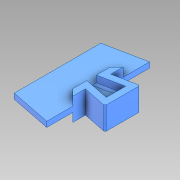
# Autodesk Inventor part: MaleDoubleSide
Saved by Autodesk Inventor 2021.4 (Build 254397000, 397)
## iProperties
Created: 2021-02-11
Part Number: MaleDoubleSide
Material: ABS プラスチック
Document SubType Name: Modeling
Designer: kumagai
Density: 1.06 g/cm^3
Appearance: 滑らか - 青
cp: 0.000 mm
ConnectorLength: 15.000 mm
RailWidth: 38.000 mm
JointFH: 9.500 mm
PrinterOffset: 0.000 mm
StraightLength: 215.000 mm
OuterWall: 2.000 mm
InnerWall: 2.400 mm
InsideWidth: 18.600 mm
RailHeight: 8.400 mm
RailDepth: 3.200 mm
JointMW1: 13.000 mm
JointMW2: 9.400 mm
JointMH: 9.000 mm
JointFW1: 13.300 mm
JointFW2: 9.600 mm
SupportGap: 0.200 mm
SupportRib: 0.650 mm
d111: 9.000 mm
d112: 2.400 mm
d113: 18.600 mm
d114: 38.000 mm
d115: 2.000 mm
d116: 13.000 mm
d117: 9.400 mm
d119: 0.000 mm
d118: 0.000 mm
d144: 0.000 mm
d143: 0.000 mm
d179: 0.500 mm
Author: kumagai
Autodesk Inventor part; units mm, degrees
ref_plane "YZ Plane" through (0, 0, 0) normal (1, 0, 0) x (0, 1, 0)
ref_plane "BackFace" through (0, -1, 0) normal (0, 1, 0) x (-1, 0, 0)
ref_plane "BottomFace" through (0, -4.2, 0) normal (0, 1, 0) x (-1, 0, 0)
sketch "FemaleOutline" plane through (0, 0, 0) normal (0, 1, 0) x (-1, 0, 0)
  line L0 (0, -26.6) -> (0, 26.6) projected
  line L1 (-3, 0) -> (18, 0) projected
  line L2 (0.4908, -4.8956) -> (9.5, -6.65)
  line L3 (9.5, -6.65) -> (9.5, 6.65)
  line L4 (9.5, 6.65) -> (0.4908, 4.8956)
  line L5 (0, -19) -> (0, -5.3)
  line L6 (0, 5.3) -> (0, 19)
  line L7 (2.4, -6.9) -> (11.5, -6.9)
  line L8 (11.5, -6.9) -> (11.5, 6.9)
  line L9 (11.5, 6.9) -> (2.4, 6.9)
  line L10 (2.4, -6.9) -> (0, -9.3)
  line L11 (2.4, 6.9) -> (0, 9.3)
  line L12 (15, -16) -> (15, 16)
  line L13 (15, 16) -> (0, 19)
  line L14 (15, -16) -> (0, -19)
  line L15 (0.4908, 4.8956) -> (0, 5.3)
  line L16 (0.4908, -4.8956) -> (0, -5.3)
  point P0 (0, 0)
  point P1 (0, -4.8)
  point P2 (0, 4.8)
  point P3 (0, 9.3)
  point P4 (0, 4.8)
  point P5 (0, -4.8)
  point P6 (0, -9.3)
  point P7 (0, -5.3)
  point P8 (0, 5.3)
  dimension "d3" = 13.3
  dimension "d5" = 9.6
  dimension "d14" = 2
  dimension "d63" = 2.4
  dimension "d64" = 18.6
  dimension "d65" = 15
  dimension "d74" = 38
  dimension "d75" = 3
  dimension "d93" = 9.5
  dimension "d94" = 2.4
  dimension "d95" = 0.5
  dimension "d96" = 0.5
  dimension "d97" = 0.5
  dimension "d98" = 0.5
  constraints: 30 end point, 6 point on line, 2 collinear, 2 horizontal, 2 vertical, 1 parallel, 1 symmetric about line, 3 other
  measures "d3" distance of L3.end L2.end
  measures "d5" distance of point (0, 4.8) point (0, -4.8)
  measures "d14" distance between parallel lines of L3 L8
  measures "d63" horizontal distance of L10.end L7.start
  measures "d64" distance of L11.end L10.end
  measures "d65" distance between parallel lines of L12 L0
  measures "d74" distance of L5.start L6.end
  measures "d75" vertical distance of L12.end L6.end
  measures "d93" distance between parallel lines of L0 L3
  measures "d94" distance from line of L0 L7.start
  measures "d95" distance of L4.end point (0, 4.8)
  measures "d96" distance of L6.start point (0, 4.8)
  measures "d97" distance of L2.start point (0, -4.8)
  measures "d98" distance of L5.end point (0, -4.8)
sketch "MaleOutline" plane through (0, 0, 0) normal (0, 1, 0) x (-1, 0, 0)
  line L0 (0, -4.7) -> (-8.5097, -6.4019)
  line L1 (-9, -6) -> (-9, 6)
  line L2 (-8.5097, 6.4019) -> (0, 4.7)
  line L3 (0, -19) -> (0, -4.7)
  line L4 (0, 4.7) -> (0, 19)
  line L5 (2.4, -1.7725) -> (-6.6, -3.5725)
  line L6 (-6.6, -3.5725) -> (-6.6, 3.5725)
  line L7 (-6.6, 3.5725) -> (2.4, 1.7725)
  line L8 (2.4, -6.9) -> (2.4, -1.7725)
  line L9 (2.4, 1.7725) -> (2.4, 6.9)
  line L10 (2.4, -6.9) -> (0, -9.3)
  line L11 (2.4, 6.9) -> (0, 9.3)
  line L12 (15, -16) -> (15, 16)
  line L13 (15, 16) -> (0, 19)
  line L14 (15, -16) -> (0, -19)
  line L15 (0, -26.6) -> (0, 26.6) projected
  line L16 (-13.8, 0) -> (19.8, 0) projected
  line L17 (-8.5097, -6.4019) -> (-9, -6)
  line L18 (-9, 6) -> (-8.5097, 6.4019)
  point P0 (-9, -6.5)
  point P1 (-9, 6.5)
  dimension "d99" = 9
  dimension "d100" = 13
  dimension "d101" = 9.4
  dimension "d102" = 2.4
  dimension "d103" = 2.4
  dimension "d104" = 2.4
  dimension "d105" = 2.4
  dimension "d106" = 2.4
  dimension "d107" = 18.6
  dimension "d109" = 38
  dimension "d110" = 3
  dimension "d120" = 15
  dimension "d128" = 0.5
  dimension "d129" = 0.5
  dimension "d130" = 0.5
  dimension "d131" = 0.5
  constraints: 34 end point, 7 point on line, 3 parallel, 2 collinear, 2 vertical, 3 other
  measures "d99" distance between parallel lines of L1 L3
  measures "d100" distance of point (-9, 6.5) point (-9, -6.5)
  measures "d101" distance of L4.start L0.start
  measures "d102" distance between parallel lines of L3 L8
  measures "d103" distance between parallel lines of L1 L6
  measures "d104" distance between parallel lines of L2 L7
  measures "d105" distance between parallel lines of L5 L0
  measures "d106" horizontal distance of L10.end L8.start
  measures "d107" distance of L11.end L10.end
  measures "d109" distance of L3.start L4.end
  measures "d110" vertical distance of L13.start L4.end
  measures "d120" distance between parallel lines of L4 L12
  measures "d128" distance of L0.end point (-9, -6.5)
  measures "d129" distance of L1.start point (-9, -6.5)
  measures "d130" distance of L1.end point (-9, 6.5)
  measures "d131" distance of L2.start point (-9, 6.5)
sketch "DipOutline" plane through (0, -1, 0) normal (0, 1, 0) x (-1, 0, 0)
  line L0 (0, -120.0212) -> (0, 93.8212) projected
  line L1 (-3, 0) -> (18, 0) projected
  line L2 (0, 19) -> (15, 16)
  line L3 (15, 16) -> (15, -16)
  line L4 (15, -16) -> (0, -19)
  line L5 (0, -19) -> (0, 19)
  line L6 (0, 19) -> (0, 4.7)
  line L7 (10.95, -6.3) -> (14.95, -6.3)
  line L8 (14.95, -6.3) -> (14.95, -2.6)
  line L9 (14.95, -2.6) -> (10.95, -2.6)
  line L10 (10.95, -2.6) -> (10.95, -6.3)
  line L11 (14.95, -15.85) -> (14.95, -10.35)
  arc A0 (14.95, -10.35) -> (0, -8.95) centre (0, -89.4723) ccw
  arc A1 (0, -17.25) -> (14.95, -15.85) centre (0, 63.2723) ccw
  line L12 (9.5, 0) -> (9.5, -6.9)
  line L13 (9.5, -6.9) -> (0, -6.9)
  line L14 (0, -8.45) -> (0.5, -8.9516)
  line L15 (0, -17.75) -> (0.5, -17.2484)
  point P0 (0, -17.25)
  point P1 (15, 0)
  point P2 (0, 0)
  point P3 (0, -8.95)
  dimension "d133" = 15
  dimension "d134" = 38
  dimension "d135" = 3
  dimension "d146" = 3.7
  dimension "d147" = 6.3
  dimension "d148" = 2.6
  dimension "d151" = 14.95
  dimension "d152" = 4
  dimension "d153" = 5.5
  dimension "d154" = 8.3
  dimension "d155" = 17.25
  dimension "d160" = 6.9
  dimension "d161" = 9.5
  dimension "d196" = 0.5
  dimension "d197" = 0.5
  dimension "d198" = 0.5
  dimension "d199" = 0.5
  constraints: 28 end point, 8 point on line, 6 point on circle, 5 vertical, 2 centre point, 2 horizontal, 2 line through centre, 2 parallel, 1 collinear, 1 equal radius, 1 other
  measures "d133" distance between parallel lines of L0 L3
  measures "d134" distance of L2.start L4.end
  measures "d135" vertical distance of L2.start L2.end
  measures "d146" distance between parallel lines of L7 L9
  measures "d147" distance between parallel lines of L1 L7
  measures "d148" distance between parallel lines of L1 L9
  measures "d151" distance between parallel lines of L8 L0
  measures "d152" distance between parallel lines of L8 L10
  measures "d153" distance of L11.end L11.start
  measures "d154" distance of A0.end A1.start
  measures "d155" distance from line of L1 A1.start
  measures "d160" distance between parallel lines of L13 L1
  measures "d161" distance between parallel lines of L5 L12
  measures "d196" distance of A0.end L14.start
  measures "d197" distance of L14.end A0.end
  measures "d198" distance of A1.start L15.end
  measures "d199" distance of A1.start L15.start
sketch "DipSupport" plane through (0, -4.2, 0) normal (0, 1, 0) x (-1, 0, 0)
  line L0 (0, -20.94) -> (0, 3.49) projected
  line L1 (-5.0794, 0) -> (17.4132, 0) projected
  line L2 (-1.8662, -13.1) -> (-0.8497, -13.1)
  line L3 (0, -9.95) -> (0, -16.25)
  line L4 (0, -16.25) -> (0.6, -16.25)
  line L5 (0.6, -16.25) -> (0.6, -15.5)
  line L6 (0.6, -14.8486) -> (0.6, -13.35)
  line L7 (0.6, -13.35) -> (13.117, -13.35)
  line L8 (13.117, -13.35) -> (13.4421, -13.9987)
  line L9 (13.4421, -13.9987) -> (0.6, -14.8486)
  line L10 (0.6, -12.85) -> (13.117, -12.85)
  line L11 (13.117, -12.85) -> (13.4421, -12.2013)
  line L12 (13.4421, -12.2013) -> (0.6, -11.3514)
  line L13 (0.6, -11.3514) -> (0.6, -12.85)
  line L14 (0, -9.95) -> (0.6, -9.95)
  line L15 (0.6, -9.95) -> (0.6, -10.7)
  line L16 (0, -9.95) -> (0, -8.75)
  line L17 (0, -8.75) -> (0.3, -8.75)
  line L18 (0.3, -8.75) -> (0.6, -9.05)
  line L19 (0.6, -9.05) -> (0.6, -9.95)
  line L20 (0, -16.25) -> (0, -17.45)
  line L21 (0.3, -17.45) -> (0.6, -17.15)
  line L22 (0.6, -17.15) -> (0.6, -16.25)
  line L23 (0, -17.45) -> (0.3, -17.45)
  line L24 (0.6, -15.5) -> (14.2, -14.6)
  line L25 (14.2, -14.6) -> (14.2, -13.9486)
  line L26 (14.2, -13.9486) -> (13.9, -13.35)
  line L27 (13.9, -13.35) -> (13.9, -12.85)
  line L28 (13.9, -12.85) -> (14.2, -12.2514)
  line L29 (14.2, -12.2514) -> (14.2, -11.6)
  line L30 (14.2, -11.6) -> (0.6, -10.7)
  line L31 (0, -9.95) -> (0, -8.75)
  line L32 (0, -16.25) -> (0, -17.45)
  point P0 (0, 0)
  point P1 (0, -17.25)
  point P2 (0, -8.95)
  dimension "d169" = 0.5
  dimension "d171" = 4.8
  dimension "d181" = 4.15
  dimension "d182" = 4.15
  dimension "d183" = 0.2
  dimension "d184" = 1
  dimension "d185" = 0.3
  dimension "d186" = 0.6
  dimension "d187" = 45
  dimension "d188" = 14.2
  dimension "d189" = 3
  dimension "d190" = 0.65
  dimension "d191" = 0.3
  dimension "d193" = 0.7
  constraints: 62 end point, 6 point on line, 5 horizontal, 5 vertical, 4 parallel, 3 perpendicular, 3 symmetric about line, 2 collinear, 12 other
  measures "d169" distance between parallel lines of L10 L7
  measures "d171" distance of L15.end L5.end
  measures "d181" distance from line of L2 point (0, -17.25)
  measures "d182" distance from line of L2 point (0, -8.95)
  measures "d183" distance from line of point (0, -17.25) L23
  measures "d184" distance from line of L4 point (0, -17.25)
  measures "d185" distance of L23.start L23.end
  measures "d186" distance of the line from the sketch origin of L13
  measures "d187" angle to the sketch x axis of L21
  measures "d188" distance of the line from the sketch origin of L29
  measures "d189" distance of L29.end L24.end
  measures "d190" distance between parallel lines of L9 L24
  measures "d191" distance between parallel lines of L29 L27
  measures "d193" distance between parallel lines of L8 L26
extrude "Female1" [suppressed]
extrude "Female2" [suppressed]
chamfer "FemaleC" [suppressed]
extrude "FemaleFill" [suppressed]
extrude "Male1" add sketch "MaleOutline" along normal mid plane 8.4 separate body contours L15 L5 L8 L10 L3 | L0 L17 L1 L16 L6 L5 L15 | L1 L18 L2 L15 L7 L6 L16 | L15 L4 L11 L9 L7
extrude "Male2" add sketch "MaleOutline" along normal mid plane 2 contours L10 L8 L5 L15 L16 L12 L14 L3 | L5 L6 L16 L15 | L16 L6 L7 L15 | L15 L7 L9 L11 L4 L13 L12 L16
chamfer "MaleC" distance 0.7 angle 45 10 edges at (2.1, 1, -2.6725) (2.1, 1, 2.6725) (6.6, 1, 0) (2.1, -1, 2.6725) (6.6, -1, 0) (2.1, -1, -2.6725) (-2.4, -1, 4.3362) (-2.4, -1, -4.3362) (-2.4, 1, 4.3362) (-2.4, 1, -4.3362)
extrude "MaleFill" [suppressed]
extrude "JointDip" [suppressed]
extrude "JointDipSup1" [suppressed]
extrude "JointDipSup2" [suppressed]
mirror "JointDipM" [suppressed]
mirror "JointDipSupM" [suppressed]
sketch "PrintTab" plane through (0, -4.2, 0) normal (0, 1, 0) x (-1, 0, 0)
  line L0 (0, -30.8) -> (0, 30.8) projected
  line L1 (-10.4076, 0) -> (1.7346, 0) projected
  line L2 (0, -19) -> (0, -17)
  line L3 (0, 17) -> (0, 19)
  line L4 (0, 19) -> (-0.8, 19)
  line L5 (0, 17) -> (-0.8, 17)
  line L6 (0, -17) -> (-0.8, -17)
  line L7 (0, -19) -> (-0.8, -19)
  line L8 (-0.8, -19) -> (-0.8, -17)
  line L9 (-0.8, 17) -> (-0.8, 19)
  arc A0 (-0.8, 19) -> (-0.8, 17) centre (-4.673, 18) ccw
  arc A1 (-0.8, -17) -> (-0.8, -19) centre (-4.673, -18) ccw
  point P0 (0, 0)
  dimension "d208" = 2
  dimension "d209" = 38
  dimension "d216" = 0.8
  dimension "d217" = 4
  constraints: 16 end point, 4 horizontal, 4 point on circle, 4 point on line, 2 centre point, 2 symmetric about line, 2 vertical, 1 collinear, 1 equal radius
  measures "d208" distance of L2.end L2.start
  measures "d209" distance of L3.end L2.start
  measures "d216" distance between parallel lines of L0 L9
  measures "d217" radius of A0
extrude "PrintTab1" [suppressed]
extrude "PrintTab2" [suppressed]
equation "\"d19\" = RailHeight"
equation "\"rib\" = 0.65"
equation "\"gap\" = 0.2"
equation "\"d118\" = 0"
equation "\"d143\" = 0"
equation "\"d178\" = 0.5"
equation "\"RailHeight\" = 8.4"
